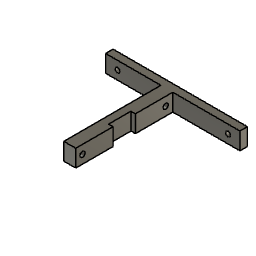
Regler_Halter_Hinten v9 (Autodesk Fusion 360 design; units mm, degrees)
Autodesk Fusion 360 part; units mm, degrees
sketch "Skizze1" plane through (0, 0, 0) normal (0, 0, 1) x (1, 0, 0)
  line L0 (0, 67) -> (45, 67)
  line L1 (45, 67) -> (45, 72)
  line L2 (45, 72) -> (-45, 72)
  line L3 (-45, 72) -> (-45, 67)
  line L4 (-45, 67) -> (-8, 67)
  line L5 (-8, 67) -> (-8, 2)
  line L6 (-8, 2) -> (0, 2)
  line L7 (0, 42) -> (-3, 42)
  line L8 (-3, 42) -> (-3, 27)
  line L9 (-3, 27) -> (0, 27)
  line L10 (0, 2) -> (0, 27)
  line L11 (0, 42) -> (0, 67)
  dimension "d1" = 5
  dimension "d2" = 5
  dimension "d3" = 65
  dimension "d4" = 8
  dimension "d7" = 15
  dimension "d8" = 3
  dimension "d9" = 25
  dimension "d22" = 45
  dimension "d35" = 45
  dimension "d36" = 80
  constraint vertical L10
  constraint perpendicular L0 L10
  constraint perpendicular L0 L1
  constraint perpendicular L2 L10
  constraint perpendicular L2 L3
  constraint perpendicular L4 L10
  constraint perpendicular L2 L5
  constraint perpendicular L6 L10
  constraint coincident L7.start L10
  constraint perpendicular L7 L10
  constraint perpendicular L7 L8
  constraint perpendicular L9 L10
  constraint collinear L10 L11
  measures "d1" distance of L2 L4
  measures "d2" distance of L0 L2
  measures "d3" distance of L6.end L0.start
  measures "d4" distance of L5 L10
  measures "d7" distance of L7.end L8.end
  measures "d8" distance of L7.start L7.end
  measures "d9" distance of L0 L7
  measures "d22" distance of L0.start L0.end
  measures "d35" distance of L3 L11
extrude "Extrusion1" add sketch "Skizze1" along normal blind 11.5
sketch "Skizze2" plane through (0, 0, 0) normal (1, 0, 0) x (0, 1, 0)
  line L0 (2, 0) -> (27, 0)
  line L1 (27, 0) -> (27, 11.5)
  line L2 (27, 11.5) -> (2, 11.5)
  line L3 (2, 11.5) -> (2, 0)
  circle A0 centre (6.5, 5.75) radius 1.75
  line L4 (67, 0) -> (67, 11.5)
  circle A1 centre (62.25, 5.75) radius 1.75
  line L5 (42, 11.5) -> (67, 11.5)
  line L6 (42, 0) -> (67, 0)
  dimension "d10" = 3.5
  dimension "d12" = 5.75
  dimension "d13" = 60.5
  dimension "d14" = 65
  dimension "d15" = 3.5
  dimension "d16" = 4.75
  dimension "d17" = 5.75
  dimension "d18" = 5.75
  measures "d10" diameter of A0
  measures "d12" distance of L2 A0.centre
  measures "d13" distance of A0.centre L4
  measures "d14" distance of L3 L4
  measures "d15" diameter of A1
  measures "d16" distance of L4 A1.centre
  measures "d17" distance of A1.centre L5
  measures "d18" distance of A1.centre L6
extrude "Extrusion2" cut sketch "Skizze2" against normal up to surface (8 mm away) contours A0 | A1
sketch "Skizze3" plane through (0, 72, 0) normal (0, 1, 0) x (-1, 0, 0)
  line L0 (-45, 0) -> (45, 0)
  line L1 (45, 0) -> (45, 11.5)
  line L2 (45, 11.5) -> (-45, 11.5)
  line L3 (-45, 11.5) -> (-45, 0)
  circle A0 centre (-37, 5.75) radius 1.6
  line L4 (-45, 11.5) -> (45, 0) construction
  line L5 (-45, 0) -> (45, 11.5) construction
  line L6 (0, 5.75) -> (0, 11.5) construction
  circle A1 centre (37, 5.75) radius 1.6
  dimension "d23" = 5.75
  dimension "d24" = 5.75
  dimension "d25" = 8
  dimension "d26" = 3.2
  constraint coincident L2.end L3.start
  constraint coincident L0.end L1.start
  constraint coincident L0.start L3.end
  constraint coincident L1.end L2.start
  constraint midpoint L5 L6.start
  constraint vertical L6
  constraint midpoint L2 L6.end
  constraint symmetric A0 L6 A1
  measures "d23" distance of L2 A0.centre
  measures "d24" distance of L0 A0.centre
  measures "d25" distance of L3 A0.centre
  measures "d26" diameter of A0
extrude "Extrusion3" cut sketch "Skizze3" against normal up to surface (5 mm away) contours A0 | A1
equation "d5 = 4 mm + 4 mm + 3.5 mm"
equation "d9 = ( 65 / 2 ) * 1 mm - ( 15 / 2 ) * 1 mm"
equation "d12 = ( ( 4 + 4 + 3.5 ) / 2 ) * 1 mm"
equation "d16 = 2.5 mm + ( 3.5 / 2 ) * 1 mm + 0.5 mm"
